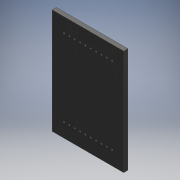
# Autodesk Inventor part: pcb
Saved by Autodesk Inventor 2016 (Build 200138000, 138)
## iProperties
Created: 2016-10-13
Part Number: pcb
Material: Generic
Document SubType Name: Modeling
Designer: Jakub
Density: 1 g/cm^3
Appearance: Default
Mass: 3.36858 g
Surface Area: 38.3025 cm^2
Volume: 3.36858 cm^3
Author: Jakub
Autodesk Inventor part; units mm, degrees
ref_plane "YZ Plane" through (0, 0, 0) normal (1, 0, 0) x (0, 1, 0)
ref_plane "XZ Plane" through (0, 0, 0) normal (0, 1, 0) x (-1, 0, 0)
sketch "Sketch1" plane through (0, 0, 0) normal (0, 1, 0) x (-1, 0, 0)
  line L0 (-17, 25) -> (17, 25)
  line L1 (17, 25) -> (17, -25)
  line L2 (17, -25) -> (-17, -25)
  line L3 (-17, -25) -> (-17, 25)
  line L4 (-17, 25) -> (17, -25) construction
  line L5 (17, 25) -> (-17, -25) construction
  point P0 (0, 0)
  dimension "d0" = 34
  dimension "d1" = 50
  constraints: 12 end point, 2 midpoint, 2 parallel, 1 horizontal, 1 perpendicular
  measures "d0" distance of L1.end L2.end
  measures "d1" distance of L0.end L1.end
extrude "Extrusion1" add sketch "Sketch1" along normal blind 2
sketch "Sketch2" plane through (0, 2, 0) normal (0, 1, 0) x (1, 0, 0)
  line L0 (17, 25) -> (-17, 25) projected
  line L1 (0, 25) -> (0, 18.3)
  line L2 (0, 18.3) -> (-1.27, 18.3)
  line L3 (-1.27, 18.3) -> (-3.81, 18.3)
  line L4 (-3.81, 18.3) -> (-6.35, 18.3)
  line L5 (-6.35, 18.3) -> (-8.89, 18.3)
  line L6 (-8.89, 18.3) -> (-11.43, 18.3)
  line L7 (0, 18.3) -> (1.27, 18.3)
  line L8 (1.27, 18.3) -> (3.81, 18.3)
  line L9 (3.81, 18.3) -> (6.35, 18.3)
  line L10 (6.35, 18.3) -> (8.89, 18.3)
  line L11 (8.89, 18.3) -> (11.43, 18.3)
  circle A0 centre (-11.43, 18.3) radius 0.5
  circle A1 centre (-8.89, 18.3) radius 0.5
  circle A2 centre (-6.35, 18.3) radius 0.5
  circle A3 centre (-3.81, 18.3) radius 0.5
  circle A4 centre (-1.27, 18.3) radius 0.5
  circle A5 centre (1.27, 18.3) radius 0.5
  circle A6 centre (3.81, 18.3) radius 0.5
  circle A7 centre (6.35, 18.3) radius 0.5
  circle A8 centre (8.89, 18.3) radius 0.5
  circle A9 centre (11.43, 18.3) radius 0.5
  point P0 (0, 0)
  dimension "d4" = 6.7
  dimension "d5" = 1.27
  dimension "d6" = 2.54
  dimension "d7" = 2.54
  dimension "d8" = 2.54
  dimension "d9" = 2.54
  dimension "d10" = 1.27
  dimension "d11" = 2.54
  dimension "d12" = 2.54
  dimension "d13" = 2.54
  dimension "d14" = 2.54
  dimension "d15" = 1
  dimension "d16" = 1
  dimension "d17" = 1
  dimension "d18" = 1
  dimension "d19" = 1
  dimension "d20" = 1
  dimension "d21" = 1
  dimension "d22" = 1
  dimension "d23" = 1
  dimension "d24" = 1
  constraints: 22 end point, 10 centre point, 10 coincident, 7 point on line, 2 horizontal, 1 midpoint, 1 perpendicular, 1 vertical
  measures "d4" distance of L1.start L1.end
  measures "d5" distance of L1.end L2.end
  measures "d6" distance of L2.end L3.end
  measures "d7" distance of L3.end L4.end
  measures "d8" distance of L4.end L5.end
  measures "d9" distance of L5.end L6.end
  measures "d10" distance of L1.end L7.end
  measures "d11" distance of L7.end L8.end
  measures "d12" distance of L8.end L9.end
  measures "d13" distance of L9.end L10.end
  measures "d14" distance of L10.end L11.end
  measures "d15" diameter of A0
  measures "d16" diameter of A1
  measures "d17" diameter of A2
  measures "d18" diameter of A3
  measures "d19" diameter of A4
  measures "d20" diameter of A5
  measures "d21" diameter of A6
  measures "d22" diameter of A7
  measures "d23" diameter of A8
  measures "d24" diameter of A9
extrude "Extrusion2" cut sketch "Sketch2" against normal up to next
ref_plane "Work Plane1" through (-17, 2, 0) normal (0, 0, 1) x (1, 0, 0)
mirror "Mirror1" about plane through (-17, 2, 0) normal (0, 0, 1) of "Extrusion2"
body "Solid1"
